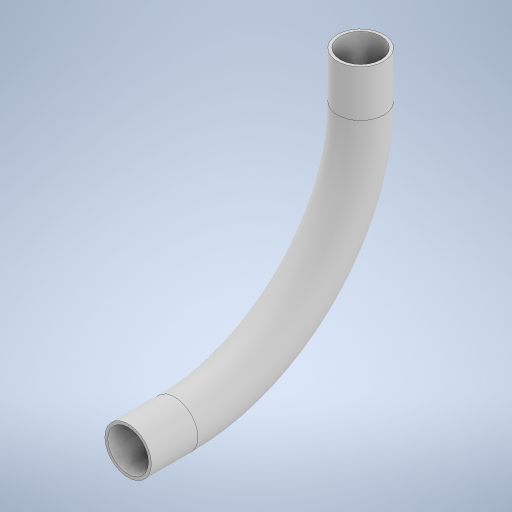
# Autodesk Inventor part: Tube Bend
Saved by Autodesk Inventor 2023 (Build 270158000, 158)
## iProperties
Created: 2023-02-03
Part Number: Tube Bend
Material: Generic
Document SubType Name: Modeling
Designer: Admin
Density: 1 g/cm^3
Appearance: Default
Author: Admin
Autodesk Inventor part; units mm, degrees
ref_plane "YZ Plane" through (0, 0, 0) normal (1, 0, 0) x (0, 1, 0)
ref_plane "XZ Plane" through (0, 0, 0) normal (0, 1, 0) x (-1, 0, 0)
ref_plane "XY Plane" through (0, 0, 0) normal (0, 0, 1) x (1, 0, 0)
sketch "Sketch1" plane through (0, 0, 0) normal (1, 0, 0) x (0, 1, 0)
  line L0 (0, 0) -> (0, -101.6)
  arc A0 (0, -101.6) -> (406.4, -508) centre (406.4, -101.6) ccw
  line L1 (406.4, -508) -> (508, -508)
  dimension "bendAngle" = 90
  dimension "centerlineRadius" = 406.4
  dimension "tangentLength" = 101.6
  constraints: 4 end point, 2 point on circle, 2 tangent, 1 centre point, 1 perpendicular, 1 vertical
  measures "bendAngle" angle of L1 L0
  measures "centerlineRadius" radius of A0
  measures "tangentLength" distance of L0.start L0.end
sketch "Sketch2" plane through (0, 0, 0) normal (0, 0, 1) x (1, 0, 0)
  circle A0 centre (0, 0) radius 50.8
  circle A1 centre (0, 0) radius 44.45
  dimension "outerDiameter" = 101.6
  dimension "wallThickness" = 6.35
  constraints: 2 centre point, 1 coincident
  measures "outerDiameter" diameter of A0
  measures "wallThickness" radial gap between concentric circles of A0 A1
sweep "Sweep1" add profiles "Sketch2" path "Sketch1"
body "Solid1"
